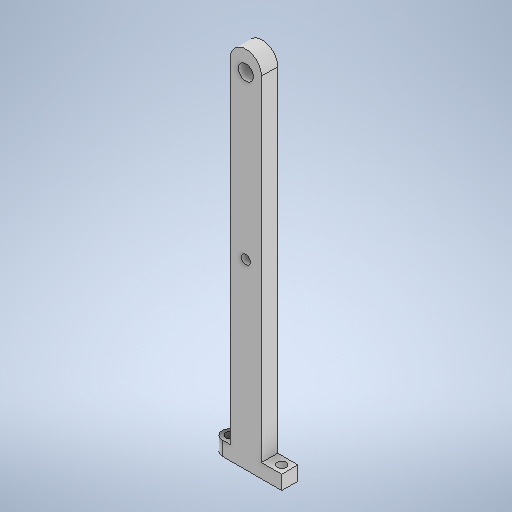
# Autodesk Inventor part: Slide Strut
Saved by Autodesk Inventor 2025 (Build 290162000, 162)
## iProperties
Created: 2024-10-25
Part Number: Slide Strut
Material: Generic
Document SubType Name: Modeling
Designer: liaco
Density: 1 g/cm^3
Appearance: Default
Author: liaco
Autodesk Inventor part; units mm, degrees
ref_plane "YZ Plane" through (0, 0, 0) normal (1, 0, 0) x (0, 1, 0)
ref_plane "XZ Plane" through (0, 0, 0) normal (0, 1, 0) x (-1, 0, 0)
ref_plane "XY Plane" through (0, 0, 0) normal (0, 0, 1) x (1, 0, 0)
sketch "Sketch1" plane through (0, 0, 0) normal (0, 0, 1) x (1, 0, 0)
  line L0 (-15.4, 0) -> (0, 0)
  line L1 (0, 0) -> (0, 180)
  line L2 (0, 180) -> (-15.4, 180)
  line L3 (-15.4, 180) -> (-15.4, 0)
  point P0 (0, 0)
  point P1 (-7.7, 170)
  dimension "d0" = 15.4
  dimension "d1" = 180
  dimension "d2" = 0
  dimension "d3" = 0
  dimension "d4" = 7.7
  dimension "d5" = 170
  constraints: 8 end point, 2 parallel, 1 horizontal, 1 perpendicular
  measures "d0" distance of L1.end L2.end
  measures "d1" distance of L0.end L1.end
  measures "d2" distance from line of L0 point (0, 0)
  measures "d3" distance from line of L1 point (0, 0)
  measures "d4" distance from line of L1 point (-7.7, 170)
  measures "d5" distance from line of L0 point (-7.7, 170)
extrude "Extrusion1" add sketch "Sketch1" along normal blind 8
hole "Hole1" at (-7.7, 170, 0) direction (0, 0, 1) diameter 7.525 end through all
sketch "Sketch2" plane through (0, 0, 0) normal (1, 0, 0) x (0, 0, -1)
  point P0 (0, 0)
sketch "Sketch5" plane through (0, 0, 0) normal (0, 0, -1) x (-1, 0, 0)
  line L0 (15.4, 180) -> (15.4, 0) projected
  line L1 (15.4, 0) -> (0, 0) projected
  point P0 (7.7, 90)
  dimension "d27" = 7.7
  dimension "d28" = 90
  measures "d27" distance from line of L0 point (7.7, 90)
  measures "d28" distance from line of L1 point (7.7, 90)
full round fillet "Full Round Fillet1" first side at (0, 60, 2.6667) centre faces at (-5.1333, 180, 2.6667) second side at (-15.4, 120, 2.6667)
hole "Hole3" at (-7.7, 90, 0) direction (0, 0, 1) diameter 4.5 end through all clearance for "Flat Head Machine Screw" size "M4" standard "Ansi Metric M Profile"
sketch "Sketch6" plane through (0, 0, 8) normal (1, 0, 0) x (0, 0, -1)
  line L0 (0, 172.3) -> (0, 0) projected
  line L1 (8, 172.3) -> (8, 0) projected
  line L2 (0, 0) -> (8, 0)
  line L3 (8, 0) -> (8, 7)
  line L4 (8, 7) -> (0, 7)
  line L5 (0, 7) -> (0, 0)
  point P0 (8, 0)
  point P1 (0, 7)
  dimension "d36" = 7
  constraints: 8 end point, 2 parallel, 1 horizontal, 1 perpendicular, 1 point on line
  measures "d36" distance between parallel lines of L2 L4
extrude "Extrusion3" add sketch "Sketch6" along normal blind 10
sketch "Sketch7" plane through (0, 7, 8) normal (0, 1, 0) x (1, 0, 0)
  line L0 (0, 8) -> (10, 8) projected
  line L1 (10, 8) -> (10, 0) projected
  point P0 (6, 4)
  dimension "d39" = 4
  dimension "d40" = 4
  measures "d39" distance from line of L0 point (6, 4)
  measures "d40" distance from line of L1 point (6, 4)
hole "Hole4" at (6, 7, 4) direction (0, -1, 0) diameter 4.5 end through all clearance for "Flat Head Machine Screw" size "M4" standard "Ansi Metric M Profile"
sketch "Sketch8" plane through (-15.4, 0, 0) normal (-1, 0, 0) x (0, 0, 1)
  point P0 (0, 0)
sketch "Sketch9" plane through (-15.4, 0, 0) normal (-1, 0, 0) x (0, 0, 1)
  line L0 (0, 0) -> (8, 0) projected
  line L1 (8, 7) -> (8, 172.3) projected
  line L2 (0, 0) -> (8, 0)
  line L3 (8, 0) -> (8, 7)
  line L4 (8, 7) -> (0, 7)
  line L5 (0, 7) -> (0, 0)
  constraints: 8 end point, 2 parallel, 1 horizontal, 1 perpendicular
extrude "Extrusion4" add sketch "Sketch9" along normal blind 8
sketch "Sketch10" plane through (-15.4, 7, 8) normal (0, 1, 0) x (1, 0, 0)
  line L0 (-8, 0) -> (-8, 8) projected
  line L1 (0, 8) -> (-8, 8) projected
  line L2 (0, 8) -> (0, 0) projected
  point P0 (15.4, 8)
  point P1 (-4, 4)
  dimension "d51" = 4
  dimension "d59" = 4
  measures "d51" distance from line of L1 point (-4, 4)
  measures "d59" distance from line of L2 point (-4, 4)
hole "Hole5" at (-19.4, 7, 4) direction (0, -1, 0) diameter 4.5 end through all clearance for "Flat Head Machine Screw" size "M4" standard "Ansi Metric M Profile"
full round fillet "Full Round Fillet2" first side at (-7.7, 33.9167, 8) centre faces at (-23.4, 2.3333, 2.6667) second side at (-7.7, 33.9167, 0)
body "Solid1"
